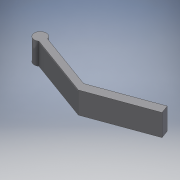
# Autodesk Inventor part: arm1
Saved by Autodesk Inventor 2020 (Build 240168000, 168)
## iProperties
Created: 2020-02-04
Part Number: arm1
Material: Generic
Document SubType Name: Modeling
Designer: Wes
Density: 1 g/cm^3
Appearance: Default
Author: Wes
Autodesk Inventor part; units mm, degrees
ref_plane "YZ Plane" through (0, 0, 0) normal (1, 0, 0) x (0, 1, 0)
ref_plane "XZ Plane" through (0, 0, 0) normal (0, 1, 0) x (-1, 0, 0)
ref_plane "XY Plane" through (0, 0, 0) normal (0, 0, 1) x (1, 0, 0)
sketch "Sketch1 - gripper" plane through (0, 0, 0) normal (0, 0, 1) x (1, 0, 0)
  line L0 (0, -65.3406) -> (0, 0) construction
  line L1 (0, 0) -> (10.2606, -28.1908)
  line L2 (10.2606, -28.1908) -> (0, -56.3816)
  line L3 (0, 0) -> (3.7588, 1.3681)
  line L4 (3.7588, 1.3681) -> (14.0194, -26.8227)
  line L5 (14.0194, -26.8227) -> (2.8794, -57.4296)
  line L6 (2.8794, -57.4296) -> (0, -56.3816)
  circle A0 centre (1.4397, -56.9056) radius 2.75
  point P0 (0.7811, -54.2356)
  point P1 (3.6605, -55.2836)
  constraints: 14 end point, 1 centre point, 1 vertical
extrude "Extrusion1" add sketch "Sketch1 - gripper" along normal blind 10
body "Solid2"
